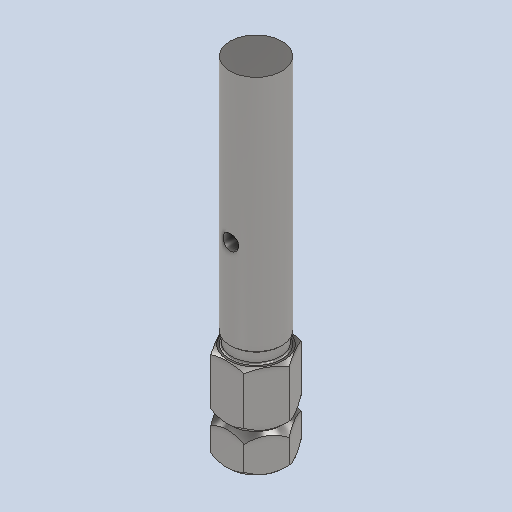
# Autodesk Inventor part: B3OFT4_HF2_kezifuro_NagyKupFogaskerekTengely
Saved by Autodesk Inventor 2023.3 (Build 273359000, 359)
## iProperties
Created: 2023-11-21
Part Number: B3OFT4_HF2_kezifuro_NagyKupFogaskerekTengely
Material: Stainless Steel
Document SubType Name: Modeling
Designer: Csábi-Kis Henrik
Density: 8 g/cm^3
Appearance: Semi-Polished
Mass: 44.2937 g
Surface Area: 24.8201 cm^2
Volume: 5.53672 cm^3
Author: Csábi-Kis Henrik
Autodesk Inventor part; units mm, degrees
ref_plane "YZ Plane" through (0, 0, 0) normal (1, 0, 0) x (0, 1, 0)
ref_plane "XZ Plane" through (0, 0, 0) normal (0, 1, 0) x (-1, 0, 0)
ref_plane "XY Plane" through (0, 0, 0) normal (0, 0, 1) x (1, 0, 0)
derived "B3OFT4_HF2_kezifuro_skeleton.ipt"
sketch "Sketch1" plane through (0, 0, 0) normal (0, 0, 1) x (1, 0, 0)
  line L0 (-14, 0) -> (14, 0) construction
  line L1 (0, 14) -> (0, -14) construction
  line L2 (-43.5, -15) -> (43.5, -15)
  line L3 (43.5, -15) -> (43.5, 15)
  line L4 (43.5, 15) -> (-43.5, 15)
  line L5 (-43.5, 15) -> (-43.5, -15)
  line L6 (-43.5, -15) -> (43.5, 15) construction
  line L7 (43.5, -15) -> (-43.5, 15) construction
  line L8 (-49.5, 21) -> (49.5, 21)
  line L9 (49.5, 21) -> (49.5, -21)
  line L10 (49.5, -21) -> (-49.5, -21)
  line L11 (-49.5, -21) -> (-49.5, 21)
  point P0 (0, 0)
sketch "Sketch2" plane through (0, 0, 0) normal (0, 1, 0) x (-1, 0, 0)
  line L0 (0, -75.2785) -> (0, 75.2785) construction
  line L1 (-69.3, 0) -> (69.3, 0) construction
  line L2 (43.5, -11) -> (-43.5, -11)
  line L3 (-43.5, -11) -> (-43.5, 11)
  line L4 (-43.5, 11) -> (43.5, 11)
  line L5 (43.5, 11) -> (43.5, -11)
  line L6 (43.5, -11) -> (-43.5, 11) construction
  line L7 (-43.5, -11) -> (43.5, 11) construction
  line L8 (22.5, 30.8) -> (-22.5, 30.8)
  line L9 (-43.5, 11) -> (-49.5, 11)
  line L10 (-49.5, 11) -> (-49.5, 0) construction
  arc A0 (-22.5, 30.8) -> (-49.5, 11) centre (-22.5, 2.4909) ccw
  line L11 (43.5, 11) -> (49.5, 11)
  arc A1 (49.5, 11) -> (22.5, 30.8) centre (22.5, 2.4909) ccw
  point P0 (43.5, 0)
  point P1 (43.5, 0)
  point P2 (43.5, 0)
  point P3 (-43.5, 0)
  point P4 (-43.5, 0)
  point P5 (-43.5, 0)
  point P6 (0, 0)
  point P7 (-49.5, 0)
  point P8 (49.5, 0)
  point P9 (49.5, 0)
  point P10 (49.5, 0)
sketch "Sketch3" plane through (0, 13, 0) normal (0, 1, 0) x (-1, 0, 0)
  line L0 (-69.3, 0) -> (69.3, 0) construction
  circle A0 centre (16.7, 0) radius 5
  circle A1 centre (-14.1, 0) radius 5
  circle A2 centre (-14.1, 0) radius 6.5
  point P0 (43.5, 0)
  point P1 (43.5, 0)
  point P2 (43.5, 0)
  point P3 (-43.5, 0)
  point P4 (-43.5, 0)
  point P5 (-43.5, 0)
sketch "Sketch4" plane through (0, 23, 0) normal (0, 1, 0) x (-1, 0, 0)
  circle A0 centre (16.7, 0) radius 5
  circle A1 centre (-14.1, 0) radius 5
sketch "Sketch5" plane through (0, -14.5, 0) normal (0, 1, 0) x (-1, 0, 0)
  circle A0 centre (16.7, 0) radius 5
  circle A1 centre (-14.1, 0) radius 5
sketch "Sketch6" plane through (0, -25, 0) normal (0, 1, 0) x (-1, 0, 0)
  circle A0 centre (16.7, 0) radius 5
  circle A1 centre (-14.1, 0) radius 5
sketch "Sketch7" plane through (0, -43, 0) normal (0, 1, 0) x (-1, 0, 0)
  line L0 (13.5246, -5.5) -> (10.3491, 0)
  line L1 (10.3491, 0) -> (13.5246, 5.5)
  line L2 (13.5246, 5.5) -> (19.8754, 5.5)
  line L3 (19.8754, 5.5) -> (23.0509, 0)
  line L4 (23.0509, 0) -> (19.8754, -5.5)
  line L5 (19.8754, -5.5) -> (13.5246, -5.5)
  point P0 (16.7, 0)
  point P1 (16.7, 0)
sketch "Sketch8" plane through (-66.5, 0, 0) normal (1, 0, 0) x (0, 1, 0)
  circle A0 centre (0, 0) radius 5
sketch "Sketch9" plane through (43.5, 0, 11) normal (0, 0, 1) x (-1, 0, 0)
  line L0 (264.4, 0) -> (-116.4, 0) construction
  line L1 (43.5, -42) -> (43.5, 91) construction
  circle A0 centre (97.5, 0) radius 2.5
  circle A1 centre (-10.5, 0) radius 2.5
  point P0 (43.5, 0)
sketch "Sketch10" plane through (42.5, 0, 0) normal (1, 0, 0) x (0, 1, 0)
  circle A0 centre (0, 0) radius 5
sketch "Sketch11" plane through (105.5, 0, 0) normal (1, 0, 0) x (0, 1, 0)
  circle A0 centre (0, 0) radius 12
  circle A1 centre (0, 0) radius 7
sketch "Sketch12" plane through (99.5, 0, 0) normal (1, 0, 0) x (0, 1, 0)
  circle A0 centre (0, 0) radius 12
  circle A1 centre (0, 0) radius 5
sketch "Sketch13" plane through (0, 0, 0) normal (0, 0, 1) x (1, 0, 0)
  line L0 (-16.7, 23) -> (-16.7, -43)
  line L1 (14.1, 23) -> (14.1, -25)
  circle A0 centre (-16.7, 2.5) radius 1.5
  circle A1 centre (14.1, 3.5) radius 1.5
  line L2 (105.5, 0) -> (30, 0)
  circle A2 centre (39, 0) radius 1.5
  line L3 (75.5, 0) -> (75.5, 15)
  line L4 (-66.5, 0) -> (-166.5, 0)
  line L5 (-11.7, -25) -> (-21.7, -25)
  line L6 (-16.7, -36) -> (-3.8491, -36)
  point P0 (42.5, 0)
  point P1 (-16.7, -27)
  point P2 (-16.7, -25)
  point P3 (-10.3491, -43)
sketch "Sketch14" plane through (30, 0, 0) normal (1, 0, 0) x (0, 1, 0)
  circle A0 centre (0, 0) radius 5
sketch "Sketch15" plane through (75.5, 15, 0) normal (0, 1, 0) x (-1, 0, 0)
  circle A0 centre (0, 0) radius 4
sketch "Sketch17" plane through (-16.7, -27, 0) normal (0, 1, 0) x (-1, 0, 0)
  circle A0 centre (0, 0) radius 11.5
  line L0 (0, 0) -> (100, 0)
  circle A1 centre (100, 0) radius 8.5
  circle A2 centre (100, 0) radius 3.5
sketch "Sketch18" plane through (0, 0, 0) normal (0, 0, 1) x (1, 0, 0)
  line L0 (-116.7, -27) -> (-116.7, -36)
  circle A0 centre (-116.7, -31.5) radius 1.5
  line L1 (-116.7, -36) -> (-116.7, -72)
sketch "Sketch19" plane through (-116.7, -72, 0) normal (0, 1, 0) x (-1, 0, 0)
  circle A0 centre (0, 0) radius 3.5
  circle A1 centre (0, 0) radius 7
sketch "Sketch20" plane through (-3.8491, -36, 0) normal (1, 0, 0) x (0, 1, 0)
  circle A0 centre (0, 0) radius 3
sketch "Sketch21" plane through (-16.7, -36, 0) normal (0, 1, 0) x (-1, 0, 0)
  circle A0 centre (0, 0) radius 5
sketch "Sketch22" plane through (-166.5, 0, 0) normal (1, 0, 0) x (0, 1, 0)
  circle A0 centre (0, 0) radius 9
  point P0 (0, 0)
ref_plane "Work Plane1" through (0, 13, 0) normal (0, 1, 0) x (-1, 0, 0)
ref_plane "Work Plane2" through (0, 23, 0) normal (0, 1, 0) x (-1, 0, 0)
ref_plane "Work Plane3" through (0, -14.5, 0) normal (0, 1, 0) x (-1, 0, 0)
ref_plane "Work Plane4" through (0, -25, 0) normal (0, 1, 0) x (-1, 0, 0)
ref_plane "Work Plane5" through (0, -43, 0) normal (0, 1, 0) x (-1, 0, 0)
ref_plane "Work Plane6" through (-66.5, 0, 0) normal (1, 0, 0) x (0, 1, 0)
ref_plane "Work Plane7" through (43.5, 0, 11) normal (0, 0, 1) x (-1, 0, 0)
ref_plane "Work Plane8" through (42.5, 0, 0) normal (1, 0, 0) x (0, 1, 0)
ref_plane "Work Plane9" through (105.5, 0, 0) normal (1, 0, 0) x (0, 1, 0)
ref_plane "Work Plane10" through (99.5, 0, 0) normal (1, 0, 0) x (0, 1, 0)
ref_plane "Work Plane11" through (30, 0, 0) normal (1, 0, 0) x (0, 1, 0)
ref_plane "Work Plane12" through (75.5, 15, 0) normal (0, 1, 0) x (-1, 0, 0)
ref_plane "Work Plane15" through (-116.7, -72, 0) normal (0, 1, 0) x (-1, 0, 0)
ref_plane "Work Plane16" through (-3.8491, -36, 0) normal (1, 0, 0) x (0, 1, 0)
ref_plane "Work Plane17" through (-16.7, -36, 0) normal (0, 1, 0) x (-1, 0, 0)
ref_plane "Work Plane20" through (0, -13.5, 0) normal (0, 1, 0) x (-1, 0, 0)
ref_plane "Work Plane21" through (0, -1.5, 0) normal (0, 1, 0) x (-1, 0, 0)
ref_plane "Work Plane22" through (37, 0, 0) normal (1, 0, 0) x (0, 1, 0)
extrude "Extrusion1" add sketch "Sketch4" against normal up to surface (48 mm away) contours A0
extrude "Extrusion2" add sketch "Sketch7" along normal up to surface (18 mm away)
sketch "Sketch23" plane through (0, 0, 0) normal (0, 0, 1) x (1, 0, 0)
  line L0 (-11.7, -36) -> (-21.7, -36) projected
  line L1 (-16.7, -36) -> (-3.8491, -36) construction
  line L2 (-11.7, -36) -> (-10.3491, -34.6491)
  line L3 (-11.7, -36) -> (-10.3491, -37.3509)
  line L4 (-10.3491, -43) -> (-10.3491, -25) projected
  line L5 (-16.7, -43) -> (-10.3491, -43) construction
  line L6 (-10.3491, -43) -> (-11.3491, -43)
  line L7 (-11.3491, -43) -> (-10.3491, -42)
  line L8 (-16.7, 23) -> (-16.7, -43) projected
  line L9 (-11.3491, -25) -> (-10.3491, -25.5774)
  line L10 (-11.3491, -25) -> (-10.3491, -25)
  line L11 (-11.7, -25) -> (-21.7, -25) projected
  line L12 (-11.7, -25) -> (-11.7, -22.7)
  line L13 (-11.7, -22.7) -> (-12, -23)
  line L14 (-12, -23) -> (-12, -25)
  dimension "d7" = 90
  dimension "d10" = 45
  dimension "d11" = 1
  dimension "d12" = 1
  dimension "d15" = 30
  dimension "d16" = 0.3
  dimension "d17" = 45
  dimension "d19" = 2
  constraints: 20 end point, 6 point on line, 2 horizontal, 1 perpendicular, 1 symmetric about line, 1 vertical
  measures "d7" angle of L3 L2
  measures "d10" angle of L5 L7
  measures "d11" distance of L4.start L6.end
  measures "d12" distance of L9.start L4.end
  measures "d15" angle of L9 L10
  measures "d16" distance between parallel lines of L12 L14
  measures "d17" angle of L12 L13
  measures "d19" distance of L13.end L14.end
revolve "Revolution1" cut sketch "Sketch23" angle 360 about axis through (-16.7, 23, 0) along (0, -1, 0)
fillet "Fillet1" radius 0.3 1 edges at (-21.4, -25, 0)
sketch "Sketch24" plane through (0, 0, 0) normal (0, 0, 1) x (1, 0, 0)
  line L0 (-16.7, 23) -> (-16.7, -43) projected
  circle A0 centre (-16.7, -5.5) radius 1.5
  dimension "d22" = 3
  dimension "d23" = 28.5
  constraints: 1 centre point, 1 point on line
  measures "d22" diameter of A0
  measures "d23" distance of L0.start A0.centre
extrude "Extrusion3" cut sketch "Sketch24" along normal through all both and the other way through all
ref_plane "Work Plane14" through (-16.7, -27, 0) normal (0, 1, 0) x (-1, 0, 0)
ref_plane "Work Plane19" through (-166.5, 0, 0) normal (1, 0, 0) x (0, 1, 0)
equation "\"d21\" = FogaskerekTengelyChamfer"
equation "\"d22\" = SzegAtmero"
equation "\"d23\" = NagyKupTengelySzegTavolsag"
equation "\"FogaskerekTengelyChamfer\" = 0.3"
equation "\"SzegAtmero\" = 3"
equation "\"NagyKupTengelySzegTavolsag\" = 28.5"
body "Solid1"
